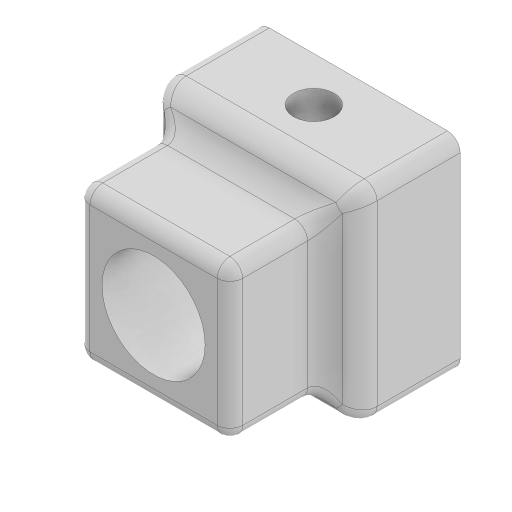
# Autodesk Inventor part: parent_ver.
Saved by Autodesk Inventor 2024 (Build 280153000, 153)
## iProperties
Created: 2023-11-07
Part Number: parent_ver.
Material: 一般
Document SubType Name: Modeling
Designer: bonju
Density: 1 g/cm^3
Appearance: 既定
Author: bonju
Autodesk Inventor part; units mm, degrees
ref_plane "YZ Plane" through (0, 0, 0) normal (1, 0, 0) x (0, 1, 0)
ref_plane "XZ Plane" through (0, 0, 0) normal (0, 1, 0) x (-1, 0, 0)
ref_plane "XY Plane" through (0, 0, 0) normal (0, 0, 1) x (1, 0, 0)
sketch "スケッチ1" plane through (0, 0, 0) normal (0, 0, 1) x (1, 0, 0)
  circle A0 centre (0, 0) radius 4.05
  line L0 (-6, 6) -> (6, 6)
  line L1 (6, 6) -> (6, -6)
  line L2 (6, -6) -> (-6, -6)
  line L3 (-6, -6) -> (-6, 6)
  line L4 (-8.4, 0) -> (8.4, 0) projected
  line L5 (0, -8.4) -> (0, 8.4) projected
  dimension "d0" = 8.1
  dimension "d19" = 12
  dimension "d20" = 12
  constraints: 8 end point, 2 parallel, 1 centre point, 1 coincident, 1 horizontal, 1 perpendicular, 2 other
  measures "d0" diameter of A0
  measures "d19" distance of L1.end L2.end
  measures "d20" distance of L0.end L1.end
extrude "押し出し1" add sketch "スケッチ1" against normal blind 8.1 contours L4 L1 L2 L5 A0 | A0 L5 L0 L1 L4 | A0 L4 L3 L0 L5 | L5 L2 L3 L4 A0
sketch "スケッチ2" plane through (0, 0, -8.1) normal (0, 0, -1) x (-1, 0, 0)
  line L0 (6, -6) -> (-6, -6) projected
  line L1 (-6, -6) -> (-6, 6) projected
  line L2 (-6, 6) -> (6, 6) projected
  line L3 (6, 6) -> (6, -6) projected
  circle A0 centre (0, 0) radius 4.05 projected
  line L4 (8, 8) -> (-8, 8)
  line L5 (-8, 8) -> (-8, -8)
  line L6 (-8, -8) -> (8, -8)
  line L7 (8, -8) -> (8, 8)
  dimension "d16" = 2
  constraints: 8 end point, 3 other
  measures "d16" distance between parallel lines of L2 L4
extrude "押し出し2" add sketch "スケッチ2" along normal blind 8 contours L0 L1 L2 L3 | A0 | L7 L6 L5 L4
sketch "スケッチ3" plane through (0, 0, 0) normal (0, 1, 0) x (-1, 0, 0)
  circle A0 centre (0, -12.6) radius 1.6
  line L0 (4.05, -8.1) -> (-4.05, -8.1) projected
  point P0 (0, 0)
  dimension "d6" = 3.2
  dimension "d7" = 4.5
  constraints: 1 centre point
  measures "d6" diameter of A0
  measures "d7" distance from line of L0 A0.centre
extrude "押し出し3" cut sketch "スケッチ3" along normal through all both and the other way through all
fillet "フィレット1" radius 2 8 edges at (0, 6, -8.1) (-6, 0, -8.1) (0, -6, -8.1) (6, 0, -8.1) (0, 8, -8.1) (8, 0, -8.1) (0, -8, -8.1) (-8, 0, -8.1)
fillet "フィレット2" radius 1 28 edges at (0, 6, 0) (0, 6, -6.1) (6, 0, -6.1) (6.2679, 6.2679, -7.1) (7.7321, 7.7321, -8.5641) (0, 8, -9.5641) (8, 0, -9.5641) (8, 8, -12.8321) (6, 6, -3.05) (-6, 0, -6.1) (-6.2679, 6.2679, -7.1) (-7.7321, 7.7321, -8.5641) (-8, 0, -9.5641) (-8, 8, -12.8321) (-6, 6, -3.05) (0, -6, -6.1) (-6.2679, -6.2679, -7.1) (-7.7321, -7.7321, -8.5641) (0, -8, -9.5641) (-8, -8, -12.8321) (-6, -6, -3.05) (6.2679, -6.2679, -7.1) (7.7321, -7.7321, -8.5641) (8, -8, -12.8321) (6, -6, -3.05) (6, 0, 0) (0, -6, 0) (-6, 0, 0)
